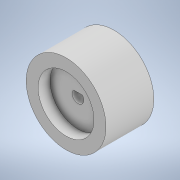
# Autodesk Inventor part: felga
Saved by Autodesk Inventor 2020.3 (Build 243373000, 373)
## iProperties
Created: 2021-03-19
Part Number: felga
Material: Ogólny
Document SubType Name: Modeling
Designer: patry
Density: 1 g/cm^3
Appearance: Domyślna
Author: patry
Autodesk Inventor part; units mm, degrees
ref_plane "YZ Plane" through (0, 0, 0) normal (1, 0, 0) x (0, 1, 0)
ref_plane "XZ Plane" through (0, 0, 0) normal (0, 1, 0) x (-1, 0, 0)
ref_plane "XY Plane" through (0, 0, 0) normal (0, 0, 1) x (1, 0, 0)
sketch "Szkic1" plane through (0, 0, 0) normal (0, 0, 1) x (1, 0, 0)
  line L0 (2.1909, 0) -> (0, 0)
  arc A0 (1.0954, -2.4) -> (2.1909, 0) centre (1.0954, -0.95) ccw
  arc A1 (0, 0) -> (1.0954, -2.4) centre (1.0954, -0.95) ccw
  circle A2 centre (1.0954, -0.95) radius 10
  point P0 (0, 0)
  dimension "d0" = 20
  constraints: 4 point on circle, 3 centre point, 2 end point, 1 coincident
  measures "d0" diameter of A2
extrude "Wyciągnięcie proste1" add sketch "Szkic1" along normal blind 9
sketch "Szkic2" plane through (1.0954, -0.95, 9) normal (0, 0, 1) x (1, 0, 0)
  circle A0 centre (0, 0) radius 10
  circle A1 centre (0, 0) radius 7
  point P0 (-1.0954, 0.95)
  dimension "d3" = 14
  dimension "d4" = 20
  constraints: 2 centre point, 1 coincident
  measures "d3" diameter of A1
  measures "d4" diameter of A0
extrude "Wyciągnięcie proste2" add sketch "Szkic2" along normal blind 3
